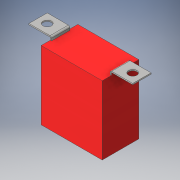
# Autodesk Inventor part: Snmubber
Saved by Autodesk Inventor 2016 (Build 200138000, 138)
## iProperties
Created: 2018-04-27
Part Number: Snmubber
Material: Generic
Document SubType Name: Modeling
Designer: Phil Erle
Density: 1 g/cm^3
Appearance: Default
Author: Phil Erle
Autodesk Inventor part; units mm, degrees
ref_plane "YZ Plane" through (0, 0, 0) normal (1, 0, 0) x (0, 1, 0)
ref_plane "XZ Plane" through (0, 0, 0) normal (0, 1, 0) x (-1, 0, 0)
ref_plane "XY Plane" through (0, 0, 0) normal (0, 0, 1) x (1, 0, 0)
sketch "Sketch1" plane through (0, 0, 0) normal (0, 0, 1) x (1, 0, 0)
  line L0 (-20, -12) -> (20, -12)
  line L1 (20, -12) -> (20, 12)
  line L2 (20, 12) -> (-20, 12)
  line L3 (-20, 12) -> (-20, -12)
  line L4 (-20, -12) -> (20, 12) construction
  line L5 (20, -12) -> (-20, 12) construction
  point P0 (0, 0)
  dimension "d0" = 40
  dimension "d1" = 24
  constraints: 12 end point, 2 midpoint, 2 parallel, 1 horizontal, 1 perpendicular
  measures "d0" distance of L1.end L2.end
  measures "d1" distance of L0.end L1.end
extrude "Extrusion1" add sketch "Sketch1" along normal blind 45
sketch "Sketch2" plane through (0, 0, 45) normal (0, 0, 1) x (1, 0, 0)
  line L0 (-20, -6) -> (-19.2, -6)
  line L1 (-19.2, -6) -> (-19.2, 6)
  line L2 (-19.2, 6) -> (-20, 6)
  line L3 (-20, 6) -> (-20, -6)
  line L4 (20, -12) -> (20, 12) projected
  line L5 (20, -6) -> (19.2, -6)
  line L6 (19.2, -6) -> (19.2, 6)
  line L7 (19.2, 6) -> (20, 6)
  line L8 (20, 6) -> (20, -6)
  point P0 (0, 0)
  point P1 (-20, 12)
  point P2 (-19.2, 0)
  point P3 (19.2, 0)
  dimension "d4" = 12
  dimension "d5" = 0.8
  dimension "d6" = 0.8
  constraints: 16 end point, 4 parallel, 3 point on line, 2 horizontal, 2 horizontal alignment, 2 midpoint, 2 perpendicular, 1 vertical alignment
  measures "d4" distance of L0.end L1.end
  measures "d5" distance of L1.end L2.end
  measures "d6" distance of L6.end L7.end
extrude "Extrusion2" add sketch "Sketch2" along normal blind 2.5
sketch "Sketch3" plane through (20, -12, 0) normal (1, 0, 0) x (0, 0, -1)
  line L0 (-47.5, 6) -> (-47.5, 18) projected
  line L1 (-47.5, 18) -> (-46.7, 18)
  line L2 (-46.7, 18) -> (-46.7, 6)
  line L3 (-46.7, 6) -> (-47.5, 6)
  line L4 (-47.5, 6) -> (-47.5, 18)
  point P0 (0, 12)
  dimension "d9" = 0.8
  constraints: 8 end point, 2 parallel, 1 horizontal, 1 perpendicular
  measures "d9" distance of L0.end L1.end
extrude "Extrusion3" add sketch "Sketch3" along normal blind 14
sketch "Sketch4" plane through (-20, -12, 0) normal (-1, 0, 0) x (0, 0, 1)
  line L0 (47.5, 18) -> (47.5, 6) projected
  line L1 (45, 18) -> (47.5, 18) projected
  line L2 (47.5, 6) -> (46.7, 6)
  line L3 (46.7, 6) -> (46.7, 18)
  line L4 (46.7, 18) -> (47.5, 18)
  line L5 (47.5, 18) -> (47.5, 6)
  point P0 (0, 12)
  dimension "d12" = 0.8
  constraints: 8 end point, 2 parallel, 1 horizontal, 1 perpendicular, 1 point on line
  measures "d12" distance between parallel lines of L0 L3
extrude "Extrusion4" add sketch "Sketch4" along normal blind 14
sketch "Sketch5" plane through (0, 0, 47.5) normal (0, 0, 1) x (1, 0, 0)
  line L0 (-28, 0) -> (28, 0) construction
  point P0 (0, 0)
  point P1 (0, 0)
  dimension "d15" = 56
  constraints: 3 coincident, 2 end point, 1 horizontal, 1 horizontal alignment, 1 midpoint
  measures "d15" distance of L0.start L0.end
hole "Hole1" at (-28, 0, 47.5) at (28, 0, 47.5) direction (0, 0, -1) diameter 5.5 end through all clearance for "Countersunk Flat Head Screw DIN EN ISO 2009" size "M5" standard "DIN"
fillet "Fillet1" radius 1 2 edges at (19.2, 0, 47.5) (-19.2, 0, 47.5)
body "Solid1"
